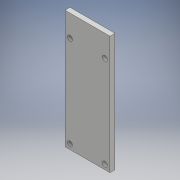
# Autodesk Inventor part: k2_t2_base
Saved by Autodesk Inventor 2017 (Build 210142000, 142)
## iProperties
Created: 2017-02-13
Part Number: k2_t2_base
Material: Generic
Document SubType Name: Modeling
Designer: herman
Density: 1 g/cm^3
Appearance: Default
Author: herman
Autodesk Inventor part; units mm, degrees
ref_plane "YZ Plane" through (0, 0, 0) normal (1, 0, 0) x (0, 1, 0)
ref_plane "XZ Plane" through (0, 0, 0) normal (0, 1, 0) x (-1, 0, 0)
ref_plane "XY Plane" through (0, 0, 0) normal (0, 0, 1) x (1, 0, 0)
sketch "Sketch1" plane through (0, 0, 0) normal (0, 1, 0) x (-1, 0, 0)
  line L0 (14.5266, 28.8729) -> (-12.4734, 28.8729)
  line L1 (-12.4734, 28.8729) -> (-12.4734, -42.1271)
  line L2 (-12.4734, -42.1271) -> (14.5266, -42.1271)
  line L3 (14.5266, -42.1271) -> (14.5266, 28.8729)
  point P0 (0, 0)
  dimension "d0" = 71
  dimension "d1" = 27
  constraints: 8 end point, 2 parallel, 1 horizontal, 1 perpendicular
  measures "d0" distance of L2.end L0.start
  measures "d1" distance of L1.end L2.end
extrude "Extrusion1" add sketch "Sketch1" along normal blind 3
sketch "Sketch2" plane through (0, 3, 0) normal (0, 1, 0) x (1, 0, 0)
  circle A0 centre (-11.5266, -15.8729) radius 1.5
  line L0 (-14.5266, -28.8729) -> (12.4734, -28.8729) projected
  line L1 (-14.5266, 42.1271) -> (-14.5266, -28.8729) projected
  circle A1 centre (-11.5266, 39.1271) radius 1.5
  circle A2 centre (9.4734, -15.8729) radius 1.5
  circle A3 centre (9.4734, 39.1271) radius 1.5
  point P0 (0, 0)
  dimension "d4" = 3
  dimension "d5" = 3
  dimension "d6" = 13
  dimension "d9" = 55
  dimension "d12" = 21
  constraints: 4 centre point, 1 horizontal, 1 vertical, 6 other
  measures "d4" diameter of A0
  measures "d5" distance from line of L1 A0.centre
  measures "d6" distance from line of L0 A0.centre
  measures "d9" distance of A0.centre A1.centre
  measures "d12" distance of A0.centre A2.centre
extrude "Extrusion2" cut sketch "Sketch2" against normal through all
body "Solid1"
